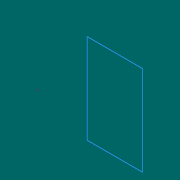
# Autodesk Inventor part: Stutze_Servo
Saved by Autodesk Inventor 2020.1 (Build 241239000, 239)
## iProperties
Created: 2020-01-27
Part Number: Stutze_Servo
Material: Generic
Document SubType Name: Modeling
Designer: Pluscrafter
Density: 1 g/cm^3
Appearance: Default
Author: Pluscrafter
Autodesk Inventor part; units mm, degrees
ref_plane "YZ Plane" through (0, 0, 0) normal (1, 0, 0) x (0, 1, 0)
ref_plane "XZ Plane" through (0, 0, 0) normal (0, 1, 0) x (-1, 0, 0)
ref_plane "XY Plane" through (0, 0, 0) normal (0, 0, 1) x (1, 0, 0)
sketch "Sketch1" plane through (0, 0, 0) normal (0, 0, 1) x (1, 0, 0)
  line L0 (46.0264, 41.778) -> (33.7264, 41.778)
  line L1 (23.7264, 31.778) -> (23.7264, -35.522)
  line L2 (56.0264, -35.522) -> (56.0264, 31.778)
  line L3 (46.0264, 32.078) -> (33.7264, 32.078)
  line L4 (33.7264, 32.078) -> (33.7264, 9.478)
  line L5 (33.7264, 9.478) -> (46.0264, 9.478)
  line L6 (46.0264, 9.478) -> (46.0264, 32.078)
  line L7 (46.0264, 32.078) -> (33.7264, 32.078) construction
  line L8 (33.7264, 32.078) -> (33.7264, 36.778) construction
  line L9 (33.7264, 36.778) -> (46.0264, 36.778) construction
  line L10 (46.0264, 36.778) -> (46.0264, 32.078) construction
  line L11 (39.8764, 36.778) -> (39.8764, 32.078) construction
  circle A0 centre (39.8764, 35.678) radius 1.1
  line L12 (46.0264, 9.478) -> (33.7264, 9.478) construction
  line L13 (33.7264, 9.478) -> (33.7264, 4.778) construction
  line L14 (33.7264, 4.778) -> (46.0264, 4.778) construction
  line L15 (46.0264, 4.778) -> (46.0264, 9.478) construction
  line L16 (39.8764, 4.778) -> (39.8764, 9.478) construction
  circle A1 centre (39.8764, 5.878) radius 1.1
  arc A2 (33.7264, 41.778) -> (23.7264, 31.778) centre (33.7264, 31.778) ccw
  arc A3 (56.0264, 31.778) -> (46.0264, 41.778) centre (46.0264, 31.778) ccw
  line L17 (34.8764, -35.522) -> (34.8764, -32.522)
  line L18 (34.8764, -32.522) -> (44.8764, -32.522)
  line L19 (44.8764, -32.522) -> (44.8764, -35.522)
  line L20 (23.7264, -35.522) -> (34.8764, -35.522)
  line L21 (44.8764, -35.522) -> (56.0264, -35.522)
  point P0 (0, 0)
  dimension "d0" = 12.3
  dimension "d1" = 22.6
  dimension "d2" = 4.7
  dimension "d3" = 1.1
  dimension "d4" = 4.7
  dimension "d5" = 1.1
  dimension "d7" = 5
  dimension "d8" = 10
  dimension "d9" = 10
  dimension "d10" = 10
  dimension "d11" = 32.3
  dimension "d12" = 10
  dimension "d13" = 11.15
  dimension "d14" = 11.15
  dimension "d17" = 45
  dimension "d18" = 45
  dimension "d20" = 42
  dimension "d21" = 12.3
  dimension "d22" = 12.3
  constraints: 44 end point, 10 parallel, 4 horizontal, 4 midpoint, 4 perpendicular, 4 point on circle, 4 tangent, 2 centre point, 2 coincident, 2 point on line, 2 vertical alignment, 1 equal radius, 4 other
  measures "d0" distance of L5.end L4.end
  measures "d1" distance between parallel lines of L5 L3
  measures "d2" distance between parallel lines of L3 L9
  measures "d3" distance from line of point (39.876, 35.678) L9
  measures "d4" distance between parallel lines of L5 L14
  measures "d5" distance from line of L14 point (39.876, 5.878)
  measures "d7" distance between parallel lines of L0 L9
  measures "d8" radius of A2
  measures "d9" distance between parallel lines of L1 L4
  measures "d10" distance between parallel lines of L2 L6
  measures "d11" distance between parallel lines of L1 L2
  measures "d12" distance of L17.end L18.end
  measures "d13" distance between parallel lines of L1 L17
  measures "d14" distance between parallel lines of L2 L19
  measures "d17" distance between parallel lines of L20 L5
  measures "d18" distance between parallel lines of L5 L21
  measures "d20" distance between parallel lines of L5 L18
  measures "d21" distance between parallel lines of L15 L13
  measures "d22" distance between parallel lines of L10 L8
extrude "Extrusion1" add sketch "Sketch1" along normal blind 3
body "Solid1"
